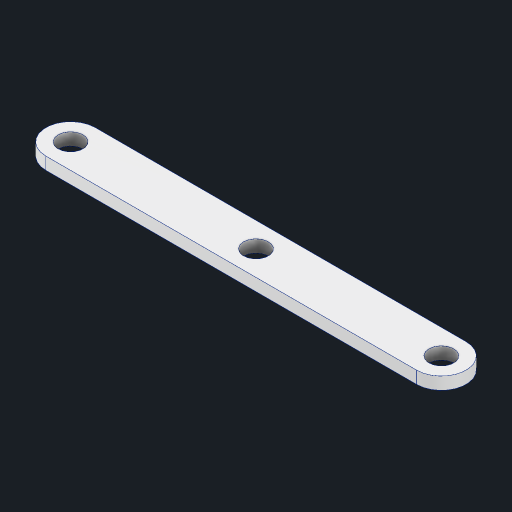
# Autodesk Inventor part: OUTK_019_PanikSiscior
Saved by Autodesk Inventor 2024.2 (Build 282272000, 272)
## iProperties
Created: 2024-12-08
Part Number: OUTK_019_PanikSiscior
Material: Aluminum 6061
Document SubType Name: Modeling
Designer: Bryan
Density: 2.7 g/cm^3
Appearance: Aluminum - Flat
Author: Bryan
Autodesk Inventor part; units mm, degrees
ref_plane "YZ Plane" through (0, 0, 0) normal (1, 0, 0) x (0, 1, 0)
ref_plane "XZ Plane" through (0, 0, 0) normal (0, 1, 0) x (-1, 0, 0)
ref_plane "XY Plane" through (0, 0, 0) normal (0, 0, 1) x (1, 0, 0)
sketch "Sketch1" plane through (0, 0, 0) normal (0, 1, 0) x (-1, 0, 0)
  circle A0 centre (0, 0) radius 3.175
  circle A1 centre (95.25, 0) radius 3.175
  line L0 (95.25, 6.35) -> (0, 6.35)
  line L1 (95.25, -6.35) -> (0, -6.35)
  line L2 (95.25, 0) -> (0, 0) construction
  arc A2 (95.25, -6.35) -> (95.25, 6.35) centre (95.25, 0) ccw
  arc A3 (0, 6.35) -> (0, -6.35) centre (0, 0) ccw
  circle A4 centre (47.625, 0) radius 3.175
  dimension "d0" = 6.35
  dimension "d1" = 6.35
  dimension "d2" = 95.25
  dimension "d3" = 12.7
  dimension "d4" = 6.35
  constraints: 6 end point, 5 centre point, 4 point on circle, 4 tangent, 3 coincident, 3 horizontal, 1 horizontal alignment, 1 midpoint
  measures "d0" diameter of A0
  measures "d1" diameter of A1
  measures "d2" distance of point (0, 0) L2.start
  measures "d3" distance between parallel lines of L1 L0
  measures "d4" diameter of A4
extrude "Extrusion1" add sketch "Sketch1" along normal blind 3.175
sketch "Sketch2" plane through (0, 3.175, 0) normal (0, 1, 0) x (1, 0, 0)
  circle A0 centre (0, 0) radius 6.35
  circle A1 centre (0, 0) radius 31.75
  dimension "d7" = 12.7
  dimension "d8" = 63.5
  constraints: 2 centre point, 2 coincident
  measures "d7" diameter of A0
  measures "d8" diameter of A1
extrude "Extrusion2" [suppressed]
sketch "Sketch3" plane through (0, 3.175, 0) normal (0, 1, 0) x (1, 0, 0)
  line L0 (-3.6662, 6.35) -> (3.6662, 6.35)
  line L1 (3.6662, 6.35) -> (7.3323, 0)
  line L2 (7.3323, 0) -> (3.6662, -6.35)
  line L3 (3.6662, -6.35) -> (-3.6662, -6.35)
  line L4 (-3.6662, -6.35) -> (-7.3323, 0)
  line L5 (-7.3323, 0) -> (-3.6662, 6.35)
  circle A0 centre (-23.8125, 0) radius 2.54
  circle A1 centre (0, 0) radius 23.8125 construction
  circle A2 centre (-11.9062, -20.6222) radius 2.54
  circle A3 centre (11.9062, -20.6222) radius 2.54
  circle A4 centre (23.8125, 0) radius 2.54
  circle A5 centre (11.9062, 20.6222) radius 2.54
  circle A6 centre (-11.9063, 20.6222) radius 2.54
  circle A7 centre (0, 0) radius 12.7
  arc A8 (-31.1085, -6.35) -> (-31.1085, 6.35) centre (0, 0) ccw projected
  line L6 (-31.1085, -6.35) -> (-2.6494, -12.4206)
  line L7 (0, 6.35) -> (-95.25, 6.35) projected
  line L8 (-31.1085, 6.35) -> (-2.6494, 12.4206)
  dimension "d13" = 47.625
  dimension "d11" = 12.7
  dimension "d12" = 5.08
  dimension "d16" = 360
  dimension "d20" = 25.4
  constraints: 16 end point, 7 centre point, 3 coincident, 2 horizontal alignment, 2 point on circle, 2 tangent, 1 horizontal, 28 other
  measures "d11" distance between parallel lines of L3 L0
  measures "d12" diameter of A0
  measures "d20" diameter of A7
extrude "Extrusion3" [suppressed]
body "Solid1"
